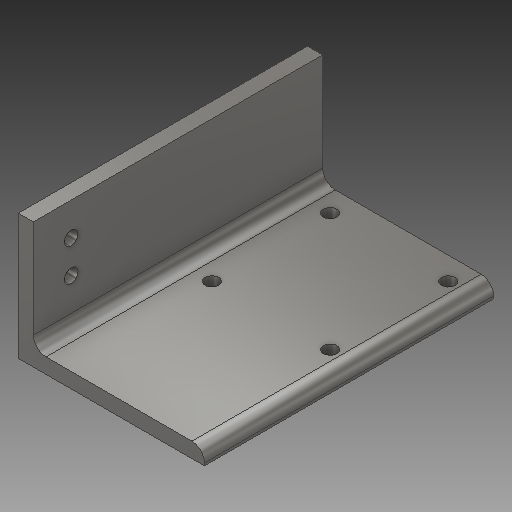
# Autodesk Inventor part: L_Fixer
Saved by Autodesk Inventor 2017 (Build 210142000, 142)
## iProperties
Created: 2016-12-12
Part Number: L_Fixer
Material: Steel, Carbon
Document SubType Name: Modeling
Designer: umr
Density: 7.85 g/cm^3
Appearance: Semi-Polished
Mass: 199.883 g
Surface Area: 104.279 cm^2
Volume: 25.4628 cm^3
Author: umr
Autodesk Inventor part; units mm, degrees
ref_plane "YZ Plane" through (0, 0, 0) normal (1, 0, 0) x (0, 1, 0)
ref_plane "XZ Plane" through (0, 0, 0) normal (0, 1, 0) x (-1, 0, 0)
sketch "Sketch1" plane through (0, 0, 0) normal (0, 1, 0) x (-1, 0, 0)
  line L0 (0, 0) -> (74, 0)
  line L1 (74, 0) -> (74, -30)
  line L2 (74, -30) -> (0, -30)
  line L3 (0, -30) -> (0, 0)
  dimension "d0" = 74
  dimension "d1" = 30
  constraints: 8 end point, 2 parallel, 1 horizontal, 1 perpendicular
  measures "d0" distance of L1.end L2.end
  measures "d1" distance of L0.end L1.end
extrude "Extrusion1" add sketch "Sketch1" along normal blind 6
fillet "Fillet1" radius 5 1 edges at (-74, 0, -15)
fillet "Fillet2" radius 5 1 edges at (0, 6, -15)
ref_plane "Work Plane1" through (-74, 0, 0) normal (0.7071, -0.7071, 0) x (0, 0, 1)
mirror "Mirror1" about plane through (-74, 0, 0) normal (0.7071, -0.7071, 0) of "Extrusion1", "Fillet2"
fillet "Fillet3" radius 5 1 edges at (-68, 6, -15)
sketch "Sketch5" plane through (0, 0, -30) normal (0, 0, -1) x (-1, 0, 0)
  line L0 (5, 6) -> (63, 6) projected
  arc A0 (5, 6) -> (0, 1) centre (5, 1) ccw projected
  line L1 (0, 0) -> (0, 1) projected
  line L2 (74, 0) -> (0, 0) projected
  line L3 (74, 0) -> (74, 74) projected
  line L4 (74, 74) -> (73, 74) projected
  arc A1 (73, 74) -> (68, 69) centre (73, 69) ccw projected
  line L5 (68, 69) -> (68, 11) projected
  arc A2 (63, 6) -> (68, 11) centre (63, 11) ccw projected
  point P0 (0, 0)
extrude "Extrusion6" add sketch "Sketch5" along normal blind 85
sketch "Sketch7" plane through (-68, 11, 0) normal (1, 0, 0) x (0, 0, -1)
  line L0 (115, 58) -> (115, 0) projected
  line L1 (115, 58) -> (115, 63) projected
  line L2 (115, -11) -> (115, 63) projected
  line L3 (0, 63) -> (115, 63) projected
  line L4 (0, 63) -> (115, 63)
  line L5 (115, 63) -> (115, 39)
  line L6 (115, 39) -> (0, 39)
  line L7 (0, 39) -> (0, 63)
  point P0 (0, -11)
  dimension "d49" = 74
  dimension "d50" = 24
  constraints: 8 end point, 2 parallel, 1 horizontal, 1 perpendicular, 1 point on line
  measures "d49" distance of L2.start L1.end
  measures "d50" distance between parallel lines of L6 L3
extrude "Extrusion7" cut sketch "Sketch7" against normal blind 10
sketch "Sketch8" plane through (-68, 11, 0) normal (1, 0, 0) x (0, 0, -1)
  circle A0 centre (15, 13) radius 2.75
  line L0 (0, 0) -> (0, 39) projected
  line L1 (115, 0) -> (0, 0) projected
  circle A1 centre (15, 26) radius 2.75
  point P0 (0, -11)
  dimension "d53" = 5.5
  dimension "d54" = 15
  dimension "d55" = 39
  dimension "d56" = 13
  dimension "d57" = 5.5
  dimension "d58" = 15
  dimension "d59" = 26
  constraints: 2 centre point
  measures "d53" diameter of A0
  measures "d54" distance from line of L0 A0.centre
  measures "d55" distance of L0.start L0.end
  measures "d56" distance from line of L1 A0.centre
  measures "d57" diameter of A1
  measures "d58" distance from line of L0 A1.centre
  measures "d59" distance from line of L1 A1.centre
extrude "Extrusion8" cut sketch "Sketch8" against normal blind 10
sketch "Sketch9" plane through (0, 0, 0) normal (0, -1, 0) x (1, 0, 0)
  line L0 (0, -115) -> (0, 0) projected
  line L1 (0, 0) -> (-74, 0) projected
  line L2 (-74, 0) -> (-74, -115) projected
  line L3 (0, -115) -> (-74, -115) projected
  circle A0 centre (-9, -106) radius 2.75
  circle A1 centre (-56, -106) radius 2.75
  circle A2 centre (-9, -59) radius 2.75
  circle A3 centre (-56, -59) radius 2.75
  dimension "d62" = 5.5
  dimension "d65" = 47
  dimension "d68" = 47
  dimension "d71" = 9
  dimension "d72" = 9
  constraints: 4 centre point, 1 horizontal, 1 vertical, 6 other
  measures "d62" diameter of A0
  measures "d65" distance of A0.centre A1.centre
  measures "d68" distance of A0.centre A2.centre
  measures "d71" distance from line of A2.centre L0
  measures "d72" distance from line of L3 A0.centre
extrude "Extrusion9" cut sketch "Sketch9" against normal blind 10 contours A0 | A1 | A2 | A3
equation "\"d56\" = 0.333333 * d55"
equation "\"d58\" = d54"
equation "\"d59\" = 2 * d56"
equation "\"d72\" = d71"
body "Solid1"
